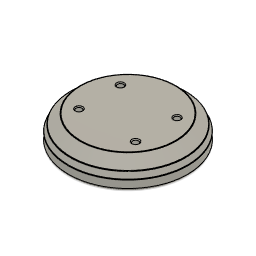
4040 Voron Z Belt Drive (Autodesk Fusion 360 archive; units mm, degrees)
design "Feet"
Autodesk Fusion 360 part; units mm, degrees
sketch "Sketch1" plane through (0, 0, 0) normal (0, 1, 0) x (1, 0, 0)
  line L0 (21.4, 19.1) -> (-21.4, 19.1)
  line L1 (-21.4, 19.1) -> (-21.4, -14.8)
  line L2 (-21.4, -14.8) -> (21.4, -14.8)
  line L3 (21.4, -14.8) -> (21.4, 19.1)
  line L4 (21.4, 19.1) -> (-21.4, -14.8) construction
  line L5 (-21.4, 19.1) -> (21.4, -14.8) construction
  circle A0 centre (0, 2.15) radius 32.5
  circle A1 centre (0, 2.15) radius 35
  line L6 (16.6, -10) -> (-16.6, -10) construction
  line L7 (-16.6, -10) -> (-16.6, 14.3) construction
  line L8 (-16.6, 14.3) -> (16.6, 14.3) construction
  line L9 (16.6, 14.3) -> (16.6, -10) construction
  line L10 (16.6, -10) -> (-16.6, 14.3) construction
  line L11 (-16.6, -10) -> (16.6, 14.3) construction
  circle A2 centre (-16.6, 14.3) radius 1.7
  circle A3 centre (16.6, 14.3) radius 1.7
  circle A4 centre (-16.6, -10) radius 1.7
  circle A5 centre (16.6, -10) radius 1.7
  point P0 (0, 2.15)
  point P1 (0, 2.15)
  dimension "d28" = 42.8
  dimension "d29" = 33.9
  dimension "d32" = 65
  dimension "d33" = 70
  dimension "d38" = 33.2
  dimension "d39" = 24.3
  dimension "d40" = 3.4
  dimension "d41" = 3.4
  dimension "d42" = 3.4
  dimension "d43" = 3.4
  constraint horizontal L0
  constraint perpendicular L0 L1
  constraint parallel L0 L2
  constraint parallel L1 L3
  constraint coincident L4 P1
  constraint coincident L5 P1
  constraint coincident P1 P0
  constraint concentric A0 A1
  constraint horizontal L6
  constraint perpendicular L6 L7
  constraint parallel L6 L8
  constraint parallel L7 L9
  constraint coincident L10 P1
  constraint coincident L11 P1
  constraint coincident L7.end L8.start
  constraint coincident L8.end L9.start
  constraint coincident L6.end L7.start
  constraint coincident L6.start L9.end
  measures "d28" distance of L1.end L2.end
  measures "d29" distance of L0.end L1.end
  measures "d32" diameter of A0
  measures "d33" diameter of A1
  measures "d38" distance of L7.end L8.end
  measures "d39" distance of L6.end L7.end
  measures "d40" diameter of A2
  measures "d41" diameter of A3
  measures "d42" diameter of A4
  measures "d43" diameter of A5
extrude "Extrude6" add sketch "Sketch1" against normal blind 10 contours L0 L1 L2 L3 | A0
extrude "Extrude7" add sketch "Sketch1" against normal blind 15 contours A1
sketch "Sketch7" plane through (0, -10, 0) normal (0, -1, 0) x (1, 0, 0)
  circle A0 centre (-16.6, 10) radius 1.7
  circle A1 centre (16.6, 10) radius 1.7
  circle A2 centre (16.6, -14.3) radius 1.7
  circle A3 centre (-16.6, -14.3) radius 1.7
  circle A4 centre (0, -2.15) radius 32.5
  circle A5 centre (16.6, 10) radius 4
  circle A6 centre (16.6, -14.3) radius 4
  circle A7 centre (-16.6, 10) radius 4
  circle A8 centre (-16.6, -14.3) radius 4
  dimension "d44" = 8
  dimension "d45" = 8
  dimension "d46" = 8
  dimension "d47" = 8
  constraint concentric A1 A5
  constraint concentric A2 A6
  constraint concentric A0 A7
  constraint concentric A3 A8
  measures "d44" diameter of A5
  measures "d45" diameter of A6
  measures "d46" diameter of A7
  measures "d47" diameter of A8
extrude "Extrude8" cut sketch "Sketch7" against normal blind 4 contours A5 | A6 | A7 | A8
chamfer "Chamfer1" distance 7 angle 45 1 edges at (-32.6315, 0, 10.5065)
fillet "Fillet4" radius 0.5 1 edges at (-26.1052, 0, -12.2752)
chamfer "Chamfer2" distance 2 angle 45 1 edges at (-32.6315, -7, 10.5065)
fillet "Fillet5" radius 1 1 edges at (-31.3129, -5.5858, -14.2951)
fillet "Fillet6" radius 1 1 edges at (-32.6315, -9, 10.5065)
fillet "Fillet7" radius 1.5 2 edges at (-32.6315, -15, -14.8065) (-30.3006, -15, 9.6025)
chamfer "Chamfer3" distance 0.5 angle 45 4 edges at (15.015, 0, -14.9147) (15.015, 0, 9.3853) (-18.185, 0, 9.3853) (-18.185, 0, -14.9147)
